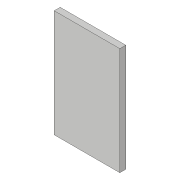
# Autodesk Inventor part: door
Saved by Autodesk Inventor 2017 (Build 210142000, 142)
## iProperties
Created: 2018-11-30
Part Number: door
Material: Generic
Document SubType Name: Modeling
Designer: jpb34
Density: 1 g/cm^3
Appearance: Default
Author: jpb34
Autodesk Inventor part; units mm, degrees
ref_plane "YZ Plane" through (0, 0, 0) normal (1, 0, 0) x (0, 1, 0)
ref_plane "XZ Plane" through (0, 0, 0) normal (0, 1, 0) x (-1, 0, 0)
ref_plane "XY Plane" through (0, 0, 0) normal (0, 0, 1) x (1, 0, 0)
sketch "Sketch1" plane through (0, 0, 0) normal (0, 0, 1) x (1, 0, 0)
  line L0 (-69.85, 114.3) -> (69.85, 114.3)
  line L1 (69.85, 114.3) -> (69.85, -114.3)
  line L2 (69.85, -114.3) -> (-69.85, -114.3)
  line L3 (-69.85, -114.3) -> (-69.85, 114.3)
  point P0 (0, 0)
  dimension "d0" = 139.7
  dimension "d1" = 228.6
  dimension "d2" = 114.3
  dimension "d3" = 69.85
  constraints: 8 end point, 2 parallel, 1 horizontal, 1 perpendicular
  measures "d0" distance of L0.start L0.end
  measures "d1" distance of L0.end L1.end
  measures "d2" distance from line of point (0, 0) L0
  measures "d3" distance from line of L1 point (0, 0)
extrude "Extrusion1" add sketch "Sketch1" along normal blind 12.7
body "Solid1"
